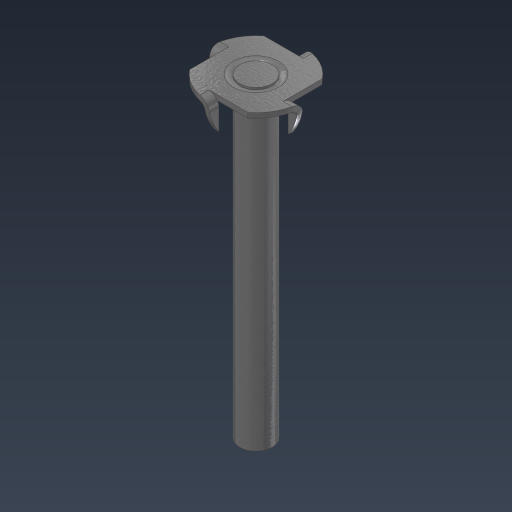
# Autodesk Inventor part: Nakrętka pazurkowa MX-01
Saved by Autodesk Inventor 2023 (Build 270158000, 158)
## iProperties
Created: 2014-02-02
Part Number: Nakrętka pazurkowa MX-01
Material: Stal, galwanizowana
Document SubType Name: Konstrukcja blachowa
Designer: Wojtek
Density: 7.85 g/cm^3
Sheet Metal Rule: Default
Mass: 2.61776 g
Surface Area: 7.7757 cm^2
Volume: 0.333472 cm^3
Appearance: Galwanizowane
Author: Wojtek
Autodesk Inventor part; units mm, degrees
ref_plane "YZ Plane" through (0, 0, 0) normal (1, 0, 0) x (0, 1, 0)
ref_plane "XZ Plane" through (0, 0, 0) normal (0, 1, 0) x (-1, 0, 0)
ref_plane "XY Plane" through (0, 0, 0) normal (0, 0, 1) x (1, 0, 0)
sketch "Szkic1" plane through (0, 0, 0) normal (1, 0, 0) x (0, 1, 0)
  line L0 (0, 0) -> (0, 6.048)
  line L1 (7.5, 8) -> (7.5, 7.2)
  line L2 (7.5, 7.2) -> (3.6, 7.2)
  line L3 (2.6, 6.2) -> (2.6, 0)
  line L4 (2.6, 0) -> (1.8, 0)
  line L5 (1.8, 0) -> (1.8, 6.2)
  line L6 (3.6, 8) -> (7.5, 8)
  arc A0 (3.6, 7.2) -> (2.6, 6.2) centre (3.6, 6.2) ccw
  arc A1 (3.6, 8) -> (1.8, 6.2) centre (3.6, 6.2) ccw
  dimension "a" = 0.8
  dimension "D" = 15
  dimension "L1" = 8
  dimension "d1" = 5.2
  dimension "r" = 1
  dimension "d6" = 1.8
  constraints: 14 end point, 5 parallel, 4 point on circle, 4 tangent, 2 centre point, 2 perpendicular, 1 horizontal alignment, 1 vertical
  measures "a" distance of L1.start L1.end
  measures "D" diameter of L1 L0
  measures "L1" distance between parallel lines of L4 L6
  measures "d1" diameter of L3 L0
  measures "r" radius of A0
  measures "d6" radius of A1
revolve "Obrót1" add sketch "Szkic1" angle 360 about axis through (0, 0, 0) along (0, 0, 1)
sketch "Szkic2" plane through (0, 0, 8) normal (0, 0, 1) x (1, 0, 0)
  circle A0 centre (0, 0) radius 7.5 projected
  line L0 (-4.6303, 5.9) -> (0, 5.9)
  line L1 (0, 5.9) -> (0, 7.5)
  dimension "d32" = 1.6
  constraints: 4 end point, 2 point on circle, 1 horizontal, 1 perpendicular, 1 vertical alignment
  measures "d32" distance of L0.end L1.end
extrude "Wyciągnięcie proste3" cut sketch "Szkic2" against normal blind 10 contours L1 L0 A0 picked at (-2.6164, 6.1914)
sketch "Szkic7" plane through (-4.6303, 5.9, 8) normal (0, 0, 1) x (1, 0, 0)
  arc A0 (0, 0) -> (4.6303, 1.6) centre (4.6303, -5.9) ccw projected
  line L0 (4.6303, 1.6) -> (4.6303, 0) projected
  line L1 (4.6303, 0) -> (5.4303, 0)
  line L2 (5.4303, 0) -> (5.4303, 1.5572)
  dimension "d20" = 0.8
  constraints: 4 end point, 1 perpendicular, 1 point on circle, 1 vertical
  measures "d20" distance of L0.end L1.end
extrude "Wyciągnięcie proste4" add sketch "Szkic7" against normal blind 5
sketch "Szkic9" plane through (0, 0, 0) normal (1, 0, 0) x (0, 1, 0)
  line L0 (7.5, 3) -> (7.5, 8) projected
  line L1 (5.9, 3) -> (7.5, 3) projected
  line L2 (0, 9.6) -> (0, -1.6) projected
  arc A0 (5.9, 3) -> (7.5, 8) centre (-1.1125, 8) ccw
  point P0 (0, 0)
  constraints: 2 point on circle, 1 centre point, 1 horizontal alignment
revolve "Obrót3" cut sketch "Szkic9" angle 360 about axis through (0, 0, 3.1) along (0, 0, -1)
fillet "Zaokrąglenie1" radius 1.6 1 edges at (0, 6.7, 8)
fillet "Zaokrąglenie2" radius 0.8 1 edges at (0.8, 6.6599, 7.2)
pattern_circular "Szyk kołowy1" count 4 over 360 about axis through (0, 0, 3.1) along (0, 0, -1) of "Wyciągnięcie proste3", "Wyciągnięcie proste4", "Zaokrąglenie1", "Zaokrąglenie2", "Obrót3"
thread "Gwint1" size "M4x0.7" class "6H" standard "ANSI Metric M Profile" full length
sketch "Sketch10" plane through (-4.6303, 5.9, 8) normal (0, 0, 1) x (1, 0, 0)
  circle A0 centre (4.6303, -5.9) radius 2.6 projected
extrude "Extrusion5" add sketch "Sketch10" against normal blind 50
equation "\"d6\" = r + a"
equation "\"d32\" = 2 * a"
equation "\"d20\" = a"
equation "\"d24\" = 2 * a"
equation "\"d25\" = a"
equation "\"Grubość\" = a"
equation "\"PromieńGięcia\" = Grubość"
equation "\"SzerokośćGięciaPodcięcia\" = Grubość"
equation "\"GłębokośćGięciaPodcięcia\" = 0.5 * Grubość"
equation "\"RozmiarPodcięciaNarożnika\" = 4 * Grubość"
equation "\"MinimalnaPozostałość\" = 2 * Grubość"
equation "\"PromieńPrzejścia\" = PromieńGięcia"
equation "\"Rozmiar_promienia_Jacobiego\" = Grubość"
equation "\"Wielk_odstępu\" = Grubość"
